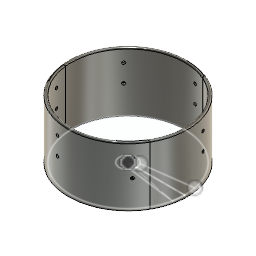
ParametricDrum (Autodesk Fusion 360 design; units mm, degrees)
Autodesk Fusion 360 part; units mm, degrees
note: some values were not read from the file. Set by a fixed rule: which face or edge a step refers to.
sketch "Sketch1" plane through (0, 0, 0) normal (0, 0, 1) x (1, 0, 0)
  arc A0 (120.7017, 39.498) -> (-0.266, 126.9997) centre (0, 0) ccw
  line L0 (0, 0) -> (120.7017, 39.498) construction
  line L1 (0, 0) -> (-0.266, 126.9997) construction
  arc A1 (117.8505, 38.565) -> (-0.2597, 123.9997) centre (0, 0) ccw
  arc A2 (114.9993, 37.632) -> (-0.2534, 120.9997) centre (0, 0) ccw
  line L2 (-0.266, 126.9997) -> (-0.2534, 120.9997)
  line L3 (120.7017, 39.498) -> (114.9993, 37.632)
  arc A3 (51.4124, 116.1282) -> (-0.266, 126.9997) centre (0, 0) ccw
  line L4 (0, 0) -> (51.4124, 116.1282) construction
  line L5 (0, 0) -> (-0.266, 126.9997) construction
  line L6 (51.4124, 116.1282) -> (48.9835, 110.6418)
  line L7 (-0.266, 126.9997) -> (2.7776, 123.9689)
  line L8 (-0.266, 126.9997) -> (-132.0155, 126.9997) construction
  line L9 (48.9835, 110.6418) -> (47.4729, 114.5527)
  arc A4 (74.8638, -102.5886) -> (120.7017, 39.498) centre (0, 0) ccw
  arc A5 (71.3269, -97.7419) -> (114.9993, 37.632) centre (0, 0) ccw
  line L10 (0, 0) -> (74.8638, -102.5886) construction
  line L11 (0, 0) -> (74.8638, -102.5886) construction
  line L12 (0, 0) -> (110.118, -63.2695) construction
  line L13 (74.8638, -102.5886) -> (75.5268, -98.3448)
  arc A6 (73.0953, -100.1652) -> (117.8505, 38.565) centre (0, 0) ccw
  line L14 (74.8638, -102.5886) -> (71.3269, -97.7419)
  line L15 (0, 0) -> (120.7017, 39.498) construction
  line L16 (104.9156, -60.2804) -> (106.0091, -64.3278)
  line L17 (74.8638, -102.5886) -> (-31.3985, -180.4748) construction
  line L18 (110.118, -63.2695) -> (104.9156, -60.2804)
  line L19 (120.7017, 39.498) -> (114.9993, 37.632)
  arc A7 (74.8638, -102.5886) -> (110.118, -63.2695) centre (0, 0) ccw
  line L20 (110.118, -63.2695) -> (105.9714, -64.3899)
  line L21 (71.3269, -97.7419) -> (75.4691, -98.3891)
  dimension "d1" = 127
  dimension "d2" = 72
  dimension "d5" = 24
  dimension "d7" = 45
  dimension "d8" = 45
  dimension "d9" = 45
  dimension "d12" = 45
  constraint coincident A0.centre L0.start
  constraint parallel L1 L2
  constraint parallel L0 L3
  constraint coincident A1.start L3
  constraint coincident A1.end L2
  constraint coincident L4 L6.end
  constraint coincident A2 L6.end
  constraint horizontal L8
  constraint coincident A1 L7.end
  constraint coincident A1 L9.end
  constraint symmetric A0.centre L3 L0.start
  constraint symmetric A0.start L3 L0.end
  constraint symmetric A0.end L3 A4.start
  constraint symmetric A0 L3 A4
  constraint symmetric A1.start L3 A6.end
  constraint symmetric A1.end L3 A6.start
  constraint symmetric A1 L3 A6
  constraint symmetric A2.start L3 A5.end
  constraint symmetric A2.end L3 A5.start
  constraint symmetric A2 L3 A5
  constraint symmetric L3 A3.start L12.end
  constraint symmetric L3 A3 A7
  constraint symmetric L3 L6.end L16.start
  constraint symmetric L3 L7.end L13.end
  constraint symmetric L3 L8.end L17.end
  constraint symmetric L3 L9.end L16.end
  constraint coincident A6 L20.end
  constraint coincident A6 L21.end
  measures "d1" radius of A0
  measures "d2" angle of L0 L1
  measures "d5" angle of L4 L5
  measures "d7" angle of L6 L9
  measures "d8" angle of L18 L20
  measures "d9" angle of L14 L21
  measures "d12" angle of L2 L7
extrude "Extrude1" add sketch "Sketch1" along normal blind 127 contours A0 A1 L3 L6 L19 | L3 A4 A6 L18 L19 | A0 A1 A3 L6 L7 | A1 A2 L3 L6 L19 | L3 A5 A6 L18 L19 | A6 L18 L20 | A1 L6 L9 | A6 L16 L18 | A5 A6 L16 L21 makes body 1
fillet "Fillet1" radius 3 2 edges at (120.3104, 12.8999, 127) (109.852, 63.7302, 127) on bodies 1
ref_plane "WorkPlane1" through (120.7017, 39.498, 0) normal (0.950407, 0.311008, 0) x (-0.311008, 0.950407, 0)
sketch "Sketch2" plane through (120.7017, 39.498, 0) normal (0.950407, 0.311008, 0) x (-0.311008, 0.950407, 0)
  line L0 (0, 124) -> (0, 98.6)
  line L1 (0, 98.6) -> (0, 60.5)
  line L2 (120.7842, 124) -> (-94.3794, 124)
  dimension "d24" = 25.4
  dimension "d25" = 38.1
  constraint vertical L0
  constraint parallel L0 L1
  constraint coincident L0.start L2
  measures "d24" distance of L0.start L0.end
  measures "d25" distance of L0.end L1.end
hole "Hole1" at (120.7017, 39.498, 98.6) at (120.7017, 39.498, 60.5) direction (-0.950407, -0.311008, 0) diameter 6.35 depth 12.7 tip angle 118 bodies 1
pattern_circular "C-Pattern2" count 6 over 360 about axis through (0, 0, 124) along (0, 0, 1) of "Hole1"
pattern_circular "C-Pattern3" count 3 over 360 about axis through (0, 0, 124) along (0, 0, 1) of bodies 1 makes body 2 at (-79.061, 99.3899, 61.5795) makes body 3 at (-46.5436, -118.1638, 61.5796)
sketch "Sketch1 (2)" plane through (0, 0, 0) normal (0, 0, 1) x (1, 0, 0) in component "Component"
  circle A0 centre (0, 0) radius 121
  circle A1 centre (0, 0) radius 18.5
  line L0 (0, 0) -> (121, 0)
  arc A2 (118.5881, -24.039) -> (121, 0) centre (0, 0) ccw
  line L1 (0, 0) -> (118.5881, -24.039) construction
  line L2 (0, 0) -> (121, 0) construction
  arc A3 (15.2687, -10.4459) -> (18.5, 0) centre (0, 0) ccw
  line L3 (0, 0) -> (15.2687, -10.4459) construction
  line L4 (0, 0) -> (18.5, 0) construction
  line L5 (118.5881, -24.039) -> (15.2687, -10.4459)
  line L6 (118.5881, 24.039) -> (15.2687, 10.4459)
  dimension "d38" = 242
  dimension "d39" = 37
  dimension "d40" = 11.459
  dimension "d41" = 34.377
  constraint coincident A0.centre A1.centre
  constraint coincident A0 L0.end
  constraint horizontal L0
  constraint coincident A1 A3.end
  constraint coincident L2 A3.end
  constraint symmetric A2.start L2 L6.start
  constraint symmetric L2 A3.start L6.end
  measures "d38" diameter of A0
  measures "d39" diameter of A1
  measures "d40" angle of L1 L2
  measures "d41" angle of L3 L4
extrude "Extrude1'" add sketch "Sketch1 (2)" along normal blind 5.08 separate body contours A0 A1 L0 L6 | A0 A1 L0 A2 A3 L5 | A1 A3 makes body 4 in component "Component"
sketch "Sketch3" plane through (0, 0, 5.08) normal (0, 0, 1) x (-1, 0, 0)
  arc A0 (-118.5881, 24.039) -> (-118.5881, -24.039) centre (0, 0) ccw
  line L0 (-118.5881, -24.039) -> (-15.2687, -10.4459)
  arc A1 (-15.2687, -10.4459) -> (-15.2687, 10.4459) centre (0, 0) ccw
  line L1 (-15.2687, 10.4459) -> (-118.5881, 24.039)
  circle A2 centre (0, 0) radius 18.5
  circle A3 centre (0, 0) radius 121
  circle A4 centre (0, 0) radius 115.92
  dimension "d44" = -5.08
extrude "Extrude2" add sketch "Sketch3" along normal blind 50.8 contours A0 L0 L1 A3 A4 bodies 4 in component "Component"
fillet "Fillet1'" offset 77 second offset 50.8 1 edges at (115.92, 0, 5.08) measured on face at (48.7307, 2.6131, 5.08) on bodies 4 in component "Component"
shell "Shell1" thickness 2.54 removed faces 2 at (3.8275, 4.8206, 5.08) at (89.9687, 2.5512, 17.8699) on bodies 4 in component "Component"
sketch "Sketch4" plane through (0, 0, 2.54) normal (0, 0, 1) x (-1, 0, 0)
  arc A0 (-116.546, 21.2084) -> (-116.546, -21.2084) centre (0, 0) ccw
  line L0 (-116.546, -21.2084) -> (-13.9723, -7.7134)
  arc A1 (-13.9723, -7.7134) -> (-13.9723, 7.7134) centre (0, 0) ccw
  line L1 (-13.9723, 7.7134) -> (-116.546, 21.2084)
  circle A2 centre (0, 0) radius 18.5
  circle A3 centre (0, 0) radius 15.96
  dimension "d51" = -2.54
extrude "Extrude3" add sketch "Sketch4" along normal blind 6.35 contours A1 A3 bodies 4 in component "Component"
fillet "Fillet2" radius 3.81 1 edges at (-15.96, 0, 5.08) on bodies 4 in component "Component"
ref_plane "WorkPlane2" through (121, 0, 27.94) normal (1, 0, 0) x (0, 1, 0)
sketch "Sketch5" plane through (121, 0, 0) normal (1, 0, 0) x (0, 1, 0)
  line L0 (0, 55.88) -> (0, 49.53)
  line L1 (0, 49.53) -> (0, 11.43)
  line L2 (0, 11.43) -> (0, 5.08)
  circle A0 centre (0, 8.255) radius 3.175
  circle A1 centre (0, 46.355) radius 3.175
  line L3 (0, 8.255) -> (-3.175, 8.255)
  line L4 (0, 8.255) -> (3.175, 8.255)
  line L5 (0, 46.355) -> (3.175, 46.355)
  line L6 (0, 46.355) -> (-3.175, 46.355)
  line L7 (3.175, 46.355) -> (3.175, 8.255)
  line L8 (-3.175, 8.255) -> (-3.175, 46.355)
  dimension "d57" = 6.35
  dimension "d58" = 38.1
  dimension "d59" = 6.35
  dimension "d60" = 6.35
  constraint vertical L0
  constraint parallel L0 L1
  constraint parallel L1 L2
  constraint coincident L2.end A0
  constraint coincident L1.end A0
  constraint coincident L0.end A1
  constraint coincident A0.centre L3.start
  constraint coincident A0 L3.end
  constraint perpendicular L2 L3
  constraint coincident A0 L4.end
  constraint perpendicular L2 L4
  constraint coincident A1.centre L5.start
  constraint coincident A1 L5.end
  constraint perpendicular L1 L5
  constraint coincident A1 L6.end
  constraint perpendicular L1 L6
  constraint tangent A0 L7
  constraint tangent A1 L8
  measures "d57" distance of L0.start L0.end
  measures "d58" distance of L0.end L1.end
  measures "d59" distance of L1.end L2.end
  measures "d60" diameter of A1
extrude "Extrude4" cut sketch "Sketch5" against normal blind 5.08 bodies 4 in component "Component"
component "Component" placed x (1, 0, 0) y (0, 1, 0) z (0, 0, 1) at (0, 0, 0)
equation "d1 = ShellDiam / 2"
equation "d2 = PieceSize * LapSize + PieceSize"
equation "d3 = -HalfShellThick"
equation "d4 = -ShellThick"
equation "d5 = PieceSize * ( LapSize * 2 )"
equation "d10 = ShellHeight"
equation "NumSegments = 3"
equation "ShellThick = 6 mm"
equation "ShellHeight = 5 in"
equation "ShellDiam = 10\""
equation "LapSize = LapSizePercent / 100"
equation "PieceSize = ( 180 / NumSegments ) * 1 deg"
equation "d22 = HalfShellThick"
equation "d24 = LugTopDist"
equation "d25 = LugSpacing"
equation "d27 = LugHoleDiam"
equation "d29 = NumSegments * 2"
equation "d31 = NumSegments"
equation "LugTopDist = 1 in"
equation "LugSpacing = 1.5 in"
equation "LapSizePercent = 20"
equation "HalfShellThick = ShellThick / 2"
equation "LugHoleDiam = 0.25 in"
equation "d38 = ShellDiam - ( ShellThick * 2 )"
equation "d40 = ( ( 360 * 1 in ) / ( PI * ShellDiam ) ) * 1 deg"
equation "d41 = ( ( 360 * 3 in ) / ( PI * ShellDiam ) ) * 1 deg"
equation "d45 = LugSpacing + ( LugHoleDiam * 2 )"
equation "d48 = ShellDiam / 2 - 50 mm"
equation "d49 = LugSpacing + ( LugHoleDiam * 2 )"
equation "d57 = LugHoleDiam"
equation "d58 = LugSpacing"
equation "d59 = LugHoleDiam"
equation "d60 = LugHoleDiam"
